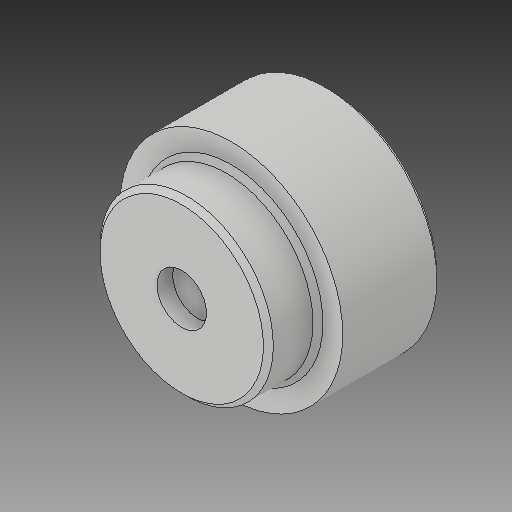
# Autodesk Inventor part: Part2
Saved by Autodesk Inventor 2019 (Build 230136000, 136)
## iProperties
Created: 2021-10-18
Part Number: Part2
Material: Generic
Document SubType Name: Modeling
Designer: Mohamed Teleb
Density: 1 g/cm^3
Appearance: Default
Mass: 41.1109 g
Surface Area: 69.9545 cm^2
Volume: 41.1109 cm^3
Author: Mohamed Teleb
Autodesk Inventor part; units mm, degrees
ref_plane "YZ Plane" through (0, 0, 0) normal (1, 0, 0) x (0, 1, 0)
ref_plane "XZ Plane" through (0, 0, 0) normal (0, 1, 0) x (-1, 0, 0)
ref_plane "XY Plane" through (0, 0, 0) normal (0, 0, 1) x (1, 0, 0)
sketch "Sketch1" plane through (0, 0, 0) normal (0, 0, 1) x (1, 0, 0)
  circle A0 centre (0, 0) radius 22.5
  dimension "d0" = 45
  constraints: 1 centre point, 1 coincident
  measures "d0" diameter of A0
extrude "Extrusion1" add sketch "Sketch1" along normal blind 20
sketch "Sketch2" plane through (0, 0, 20) normal (0, 0, 1) x (1, 0, 0)
  circle A0 centre (0, 0) radius 17.5
  dimension "d3" = 35
  constraints: 1 centre point, 1 coincident
  measures "d3" diameter of A0
extrude "Extrusion2" add sketch "Sketch2" along normal blind 10
chamfer "Chamfer1" distance 1 angle 45 1 edges at (-17.5, 0, 20)
chamfer "Chamfer2" distance 1 angle 45 1 edges at (-17.5, 0, 30)
chamfer "Chamfer3" distance 1 angle 45 1 edges at (-22.5, 0, 0)
sketch "Sketch3" plane through (0, 0, 30) normal (0, 0, 1) x (1, 0, 0)
  circle A0 centre (0, 0) radius 5
  dimension "d15" = 10
  constraints: 1 centre point, 1 coincident
  measures "d15" diameter of A0
extrude "Extrusion3" cut sketch "Sketch3" against normal blind 3.2
body "Solid1"
